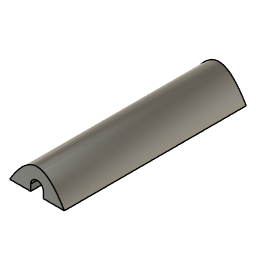
Cable Clamp (Autodesk Fusion 360 design; units mm, degrees)
Autodesk Fusion 360 part; units mm, degrees
sketch "Sketch1" plane through (0, 0, 0) normal (0, 1, 0) x (1, 0, 0)
  line L0 (0, 0) -> (6, 0)
  line L1 (3, 0) -> (3, -0.7)
  circle A0 centre (3, -0.7) radius 0.7
  line L2 (3, -0.7) -> (3, -2.7)
  spline S0 degree 5 poles (0, 0) (0.12, -0.2048) (0.36, -0.5965) (0.72, -1.1304) (1.2, -1.7331) (1.8, -2.2925) (2.4, -2.6403) (3, -2.7594) (3.6, -2.6403) (4.2, -2.2925) (4.8, -1.7331) (5.28, -1.1304) (5.64, -0.5965) (5.88, -0.2048) (6, 0) knots 0 0 0 0 0 0 0.1 0.2 0.3 0.4 0.5 0.6 0.7 0.8 0.9 1 1 1 1 1 1
  line L3 (3, -0.7) -> (2.3, -0.7)
  line L4 (2.3, -0.7) -> (2.3, 0)
  line L5 (3, -0.7) -> (3.7, -0.7)
  line L6 (3.7, -0.7) -> (3.7, 0)
  dimension "d1" = 6
  dimension "d2" = 0.7
  dimension "d3" = 2
  constraint coincident L0.start S0.start
  constraint horizontal L0
  constraint midpoint L0 L1.start
  constraint perpendicular L0 L1
  constraint coincident L1.end A0.centre
  constraint coincident L1.start A0
  constraint perpendicular L0 L2
  constraint coincident A0 L3.end
  constraint perpendicular L2 L3
  constraint coincident L0 L4.end
  constraint tangent A0 L4
  constraint coincident A0 L5.end
  constraint perpendicular L1 L5
  constraint coincident L0 L6.end
  constraint tangent A0 L6
  measures "d1" distance of L0.start L0.end
  measures "d2" distance of L1.start L1.end
  measures "d3" distance of L1.end L2.end
extrude "Extrude1" add sketch "Sketch1" along normal blind 20 contours L0 A0 L2 S0 L4 | L0 A0 L2 S0 L6
